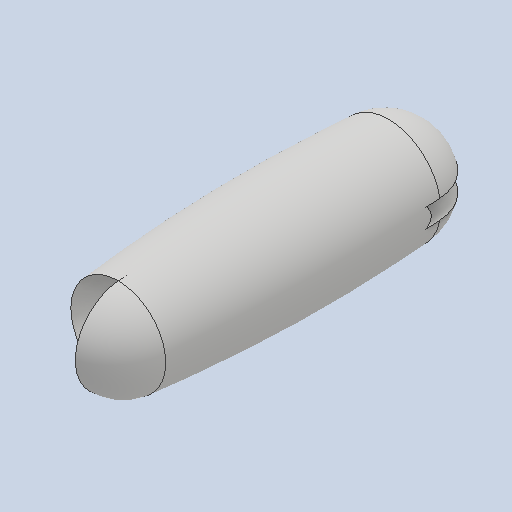
# Autodesk Inventor part: ч ASY human dummy 01
Saved by Autodesk Inventor 2025 (Build 290162010, 162A)
## iProperties
Created: 2018-05-22
Part Number: ч ASY human dummy 01
Material: Типовые
Document SubType Name: Modeling
Designer: admin
Density: 1 g/cm^3
Appearance: По умолчанию
Author: admin
Autodesk Inventor part; units mm, degrees
ref_plane "YZ Plane" through (0, 0, 0) normal (1, 0, 0) x (0, 1, 0)
ref_plane "XZ Plane" through (0, 0, 0) normal (0, 1, 0) x (-1, 0, 0)
ref_plane "XY Plane" through (0, 0, 0) normal (0, 0, 1) x (1, 0, 0)
sketch "Эскиз1" plane through (0, 0, 0) normal (0, 0, 1) x (1, 0, 0)
  arc A0 (0, 55) -> (0, -55) centre (0, 0) ccw
  line L0 (0, 55) -> (0, -55)
  dimension "d0" = 55
  constraints: 2 coincident, 2 end point, 2 point on circle, 1 centre point, 1 midpoint, 1 vertical
  measures "d0" radius of A0
revolve "Вращение1" add sketch "Эскиз1" angle 360 about axis through (0, 55, 0) along (0, -1, 0)
sketch "Эскиз2" plane through (0, 0, 0) normal (1, 0, 0) x (0, 1, 0)
  line L0 (0, -10) -> (0, 10)
  line L1 (0, -10) -> (56, -10)
  line L2 (56, -10) -> (56, 10)
  line L3 (56, 10) -> (0, 10)
  point P0 (0, 0)
  point P1 (0, 0)
  dimension "d2" = 20
  dimension "d3" = 56
  constraints: 8 end point, 2 coincident, 2 perpendicular, 1 horizontal, 1 midpoint, 1 vertical
  measures "d2" distance of L1.end L2.end
  measures "d3" distance of L2.end L0.end
sketch "Эскиз3" plane through (0, 0, 0) normal (1, 0, 0) x (0, 1, 0)
  arc A0 (-325, 0) -> (-225, 0) centre (-275, 0) ccw
  line L0 (-225, 0) -> (-325, 0)
  point P0 (0, 0)
  dimension "d5" = 275
  dimension "d6" = 50
  constraints: 2 end point, 2 horizontal alignment, 2 point on circle, 1 centre point, 1 horizontal, 1 midpoint
  measures "d5" distance of A0.centre point (0, 0)
  measures "d6" radius of A0
revolve "Вращение3" add sketch "Эскиз3" angle 180 about axis through (0, -225, 0) along (0, -1, 0)
sketch "Эскиз4" plane through (0, 0, 0) normal (0, 0, 1) x (1, 0, 0)
  line L0 (0, -325) -> (0, -225) construction
  line L1 (0, -325) -> (0, -225)
  line L2 (0, 5) -> (0, -225)
  arc A0 (49.749372, -280) -> (54.887665, 3.513433) centre (-1671.578894, -107) ccw
  line L3 (54.791865, 5) -> (0, 5) construction
  line L4 (49.749372, -280) -> (0, -280) construction
  arc A1 (0, -55) -> (54.887665, 3.513433) centre (0, 0) ccw
  arc A2 (49.749372, -280) -> (0, -225) centre (0, -275) ccw
  arc A3 (0, -325) -> (49.749372, -280) centre (0, -275) ccw construction
  arc A4 (0, -225) -> (0, -325) centre (0, -275) ccw construction
  arc A5 (54.772256, 5) -> (-54.772256, 5) centre (0, 0) ccw construction
  arc A6 (-54.772256, 5) -> (0, -55) centre (0, 0) ccw
  arc A7 (54.887665, 3.513433) -> (54.772256, 5) centre (0, 0) ccw construction
  point P0 (0, -128.982251)
  dimension "d10" = 5
  dimension "d11" = 110
  dimension "d12" = 5
  constraints: 16 point on circle, 8 centre point, 7 end point, 5 point on line, 2 coincident, 2 tangent, 1 horizontal, 1 perpendicular, 1 vertical
  measures "d10" distance from line of point (0, 0) L3
  measures "d11" diameter of A1
  measures "d12" distance from line of L4 point (0, -275)
revolve "Вращение4" add sketch "Эскиз4" angle 360 about axis through (0, 5, 0) along (0, -1, 0)
revolve "Вращение5" cut sketch "Эскиз2" angle 360 about axis through (0, 0, -10) along (0, 0, 1)
equation "\"d0\" = Shoulder_width"
equation "\"d5\" = shoulder_height"
equation "\"d11\" = 2 * Shoulder_width"
equation "\"shoulder_height\" = 275"
equation "\"Shoulder_width\" = 55"
